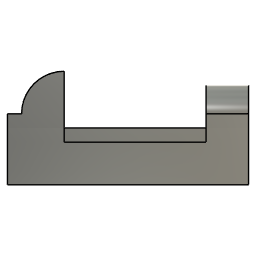
task1 B robocon (Autodesk Fusion 360 design; units mm, degrees)
Autodesk Fusion 360 part; units mm, degrees
sketch "Sketch1" plane through (0, 0, 0) normal (0, 0, 1) x (1, 0, 0)
  line L0 (3.5, -5) -> (-3.5, -5)
  line L1 (-3.5, -5) -> (-3.5, 5)
  line L2 (-3.5, 5) -> (3.5, 5)
  line L3 (3.5, 5) -> (3.5, -5)
  dimension "d1" = 7
  dimension "d2" = 10
  constraint horizontal L0
  constraint perpendicular L0 L1
  constraint parallel L0 L2
  constraint parallel L1 L3
  measures "d1" distance of L1.end L2.end
  measures "d2" distance of L0.end L1.end
extrude "Extrude1" add sketch "Sketch1" along normal blind 3 makes body 1
sketch "Sketch2" plane through (0, 0, 3) normal (0, 0, 1) x (-1, 0, 0)
  line L0 (-3.5, -5) -> (3.5, -5)
  line L1 (3.5, -5) -> (3.5, 5)
  line L2 (3.5, 5) -> (-3.5, 5)
  line L3 (-3.5, 5) -> (-3.5, -5)
  line L4 (3.5, 5) -> (-3.5, 5)
  line L5 (-3.5, 5) -> (-3.5, 9)
  line L6 (-3.5, 9) -> (3.5, 9)
  line L7 (3.5, 9) -> (3.5, 5)
  dimension "d5" = 7
  dimension "d6" = 4
  constraint horizontal L4
  constraint vertical L5
  constraint horizontal L6
  constraint vertical L7
  constraint coincident L1.end L2.start
  measures "d5" distance of L1.end L2.end
  measures "d6" distance of L1.end L6.end
extrude "Extrude2" add sketch "Sketch2" along normal blind 2 and the other way blind 3 contours L2 L4 L5 L6 L7 bodies 1
sketch "Sketch4" plane through (3.5, 0, 0) normal (1, 0, 0) x (0, 1, 0)
  line L0 (-9, 0) -> (5, 0)
  line L1 (5, 0) -> (5, 3)
  line L2 (5, 3) -> (-5, 3)
  line L3 (-5, 3) -> (-5, 5)
  line L4 (-5, 5) -> (-9, 5)
  line L5 (-9, 5) -> (-9, 0)
  line L6 (-5, 5) -> (-5, 8)
  arc A0 (-9, 0.8769) -> (-4.2583, 3) centre (-8, 5) ccw
  arc A1 (-5, 8) -> (-8, 5) centre (-5, 5) ccw
  arc A2 (-5, 2) -> (-2.7639, 3) centre (-5, 5) ccw
  dimension "d11" = 3
  dimension "d12" = 6
  constraint coincident L3.end L4.start
  constraint perpendicular L4 L6
  constraint coincident L4 A0.centre
  constraint coincident L5 A0.start
  constraint coincident L2 A0.end
  constraint coincident L2 A2.end
  constraint coincident A0 A2.start
  constraint concentric A1 A2
  measures "d11" distance of L3.end L6.end
  measures "d12" diameter of A1
extrude "Extrude3" add sketch "Sketch4" against normal blind 7 contours L4 L6 A1 bodies 1
extrude "Extrude4" add 1 faces at (3.5, -3, 1) along direction (1, 0, 0) blind 1 on bodies 1 bodies 1
sketch "Sketch6" plane through (0, -9, 0) normal (0, -1, 0) x (1, 0, 0)
  line L0 (4.5, 5) -> (-3.5, 5)
  line L1 (-3.5, 5) -> (-3.5, 0)
  line L2 (-3.5, 0) -> (4.5, 0)
  line L3 (4.5, 0) -> (4.5, 5)
  line L4 (0.5, 5) -> (0.5, 4) construction
  line L5 (-3.5, 4) -> (-0.5, 4) construction
  line L6 (-0.5, 4) -> (1.5, 4)
  line L7 (1.5, 4) -> (1.5, 2)
  line L8 (-0.5, 4) -> (-0.5, 2)
  line L9 (-0.5, 2) -> (-1.5, 2)
  line L10 (-1.5, 2) -> (-1.5, 0)
  line L11 (1.5, 2) -> (2.5, 2)
  line L12 (2.5, 2) -> (2.5, 0)
  constraint midpoint L0 L4.start
  constraint perpendicular L0 L4
  constraint coincident L1 L5.start
  constraint perpendicular L1 L5
  constraint parallel L5 L6
  constraint perpendicular L6 L7
  constraint perpendicular L6 L8
  constraint perpendicular L8 L9
  constraint coincident L2 L10.end
  constraint perpendicular L2 L10
  constraint perpendicular L7 L11
  constraint coincident L2 L12.end
  constraint perpendicular L2 L12
extrude "Extrude5" cut sketch "Sketch6" against normal blind 4 contours L2 L6 L7 L8 L9 L10 L11 L12 bodies 1
sketch "Sketch7" plane through (0, 0, 3) normal (0, 0, 1) x (-1, 0, 0)
  line L0 (-4.5, -5) -> (3.5, -5)
  line L1 (3.5, -5) -> (3.5, 5)
  line L2 (3.5, 5) -> (0.5, 5)
  line L3 (0.5, 5) -> (-1.5, 5)
  line L4 (-1.5, 5) -> (-4.5, 5)
  line L5 (-4.5, 5) -> (-4.5, -5)
  line L6 (-4.5, -5) -> (-4.5, -8)
  line L7 (-4.5, -8) -> (3.5, -8)
  line L8 (3.5, -8) -> (3.5, -5)
  dimension "d22" = 8
  constraint coincident L0.start L5.end
  constraint perpendicular L0 L6
  constraint perpendicular L6 L7
  constraint coincident L0.end L1.start
  constraint perpendicular L0 L8
  measures "d22" distance of L6.end L7.end
extrude "Extrude6" add sketch "Sketch7" along normal blind 2 and the other way blind 3 contours L0 L6 L7 L8 bodies 1
sketch "Sketch8" plane through (0, 5, 0) normal (0, -1, 0) x (1, 0, 0)
  line L0 (-3.5, 3) -> (4.5, 3)
  line L1 (4.5, 3) -> (4.5, 5)
  line L2 (4.5, 5) -> (-3.5, 5)
  line L3 (-3.5, 5) -> (-3.5, 3)
  arc A0 (2.5, 5) -> (-1.5, 5) centre (0.5, 5) ccw
  dimension "d27" = 4
  constraint midpoint L2 A0.centre
  constraint coincident L2 A0.end
  constraint coincident L2 A0.start
  measures "d27" diameter of A0
extrude "Extrude7" add sketch "Sketch8" against normal blind 3 contours L2 A0 bodies 1
sketch "Sketch9" plane through (0, -5, 0) normal (0, 1, 0) x (-1, 0, 0)
  line L0 (0.5, 4) -> (0.5, 3)
  line L1 (0.5, 3) -> (3.5, 3)
  line L2 (3.5, 3) -> (3.5, 8)
  line L3 (3.5, 8) -> (-4.5, 8)
  line L4 (-4.5, 8) -> (-4.5, 3)
  line L5 (-4.5, 3) -> (-1.5, 3)
  line L6 (-1.5, 3) -> (-1.5, 4)
  line L7 (-1.5, 4) -> (0.5, 4)
  line L8 (-1.5, 4) -> (-1.5, 3)
  line L9 (-1.5, 3) -> (0.5, 3)
  line L10 (0.5, 3) -> (0.5, 4)
  line L11 (0.5, 4) -> (-1.5, 4)
  constraint coincident L6.end L7.start
  constraint coincident L5.end L6.start
  constraint coincident L0.end L1.start
  constraint coincident L0.start L7.end
extrude "Extrude8" add sketch "Sketch9" along normal blind 10 contours L0 L6 L7 L8 L9 L10 L11 bodies 1
extrude "Extrude9" cut 1 faces at (0.8333, -5, 0.6667) along direction (0, 1, 0) blind 14 on bodies 1 bodies 1
sketch "Sketch10" plane through (0, -5, 0) normal (0, 1, 0) x (-1, 0, 0)
  line L0 (0.5, 4) -> (0.5, 3)
  line L1 (0.5, 3) -> (3.5, 3)
  line L2 (3.5, 3) -> (3.5, 8)
  line L3 (3.5, 8) -> (-4.5, 8)
  line L4 (-4.5, 8) -> (-4.5, 3)
  line L5 (-4.5, 3) -> (-1.5, 3)
  line L6 (-1.5, 3) -> (-1.5, 4)
  line L7 (-1.5, 4) -> (0.5, 4)
  line L8 (-1.5, 4) -> (0.5, 4)
  line L9 (0.5, 3) -> (-1.5, 3)
  constraint coincident L6.end L7.start
  constraint coincident L0.start L7.end
  constraint coincident L0.end L1.start
  constraint coincident L5.end L6.start
extrude "Extrude10" add sketch "Sketch10" along normal blind 10 separate body contours L0 L6 L7 L8 L9 makes body 2
